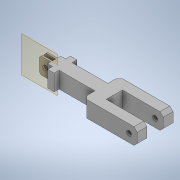
# Autodesk Inventor part: finger
Saved by Autodesk Inventor 2021 (Build 250183000, 183)
## iProperties
Created: 2020-11-29
Part Number: finger
Material: Generic
Document SubType Name: Modeling
Designer: awitc
Density: 1 g/cm^3
Appearance: Smooth - Medium Gray
Author: awitc
Autodesk Inventor part; units mm, degrees
ref_plane "YZ Plane" through (0, 0, 0) normal (1, 0, 0) x (0, 1, 0)
ref_plane "XZ Plane" through (0, 0, 0) normal (0, 1, 0) x (-1, 0, 0)
ref_plane "Work Plane1" through (0, 0, -10) normal (0, 0, 1) x (1, 0, 0)
sketch "Sketch12" plane through (0, 0, 0) normal (0, 1, 0) x (-1, 0, 0)
  line L0 (5, 4) -> (2, 4)
  line L1 (-2, 4) -> (-2, 7)
  line L2 (-2, 7) -> (2, 7)
  line L3 (2, 7) -> (2, 4)
  line L4 (6, 1) -> (12, 1)
  line L5 (12, -1) -> (6, -1)
  line L6 (12, -1) -> (6, -1)
  line L7 (6, -2) -> (12, -2)
  line L8 (5, -4) -> (5, 4)
  line L9 (12, -2) -> (12, -1)
  line L10 (12, 1) -> (12, 2)
  line L11 (12, 2) -> (6, 2)
  line L12 (6, -2) -> (5, -2)
  line L13 (6, -1) -> (5, -1)
  line L14 (6, 1) -> (5, 1)
  line L15 (6, 2) -> (5, 2)
  line L16 (-31, -11) -> (-57, -11)
  line L17 (-57, -11) -> (-57, -5)
  line L18 (-31, 11) -> (-57, 11)
  line L19 (-57, 11) -> (-57, 5)
  line L20 (-31, -11) -> (-24, -11)
  line L21 (-24, -11) -> (-24, -4)
  line L22 (-24, -4) -> (-24, 11)
  line L23 (-24, 11) -> (-31, 11)
  line L24 (-32, -4) -> (-32, 4)
  line L25 (-32, 4) -> (-32, 5)
  line L26 (-32, 5) -> (-57, 5)
  line L27 (-32, -4) -> (-32, -5)
  line L28 (-32, -5) -> (-57, -5)
  line L29 (5, -4) -> (2, -4)
  line L30 (2, -4) -> (2, -7)
  line L31 (2, -7) -> (-2, -7)
  line L32 (-2, -7) -> (-2, -4)
  line L33 (-2, -4) -> (-5, -4)
  line L34 (-5, -4) -> (-5, 4)
  line L35 (-5, 4) -> (-2, 4)
  line L36 (-5, 4) -> (-24, 4)
  line L37 (-5, -4) -> (-24, -4)
  point P0 (0, 0)
  point P1 (-31, 4)
  dimension "d118" = 4
  dimension "d156" = 7
  dimension "d170" = 3
  dimension "d171" = 3
  constraints: 76 end point, 14 perpendicular, 10 point on line, 4 horizontal, 4 vertical, 3 parallel, 1 collinear
  measures "d118" distance of L1.end L2.end
  measures "d156" distance of point (-31, 4) L18.start
  measures "d170" distance of L29.end L30.end
  measures "d171" distance of L32.end L33.end
ref_plane "Work Plane3" through (-12, 0, 2) normal (0, 0, 1) x (1, 0, 0)
extrude "Extrusion16" add sketch "Sketch12" along normal mid plane 10
extrude "Extrusion17" add sketch "Sketch12" along normal mid plane 8 contours L15 L11 L10 L4 L14 L8 | L13 L5 L9 L7 L12 L8
sketch "Sketch17" plane through (-12, 4, 2) normal (0, 0, 1) x (1, 0, 0)
  line L0 (7, -9) -> (7, 1) projected
  line L1 (7, -8) -> (3.5, -8)
  line L2 (0, -8) -> (7, -8) projected
  circle A0 centre (3.5, -4) radius 1.5
  point P0 (12, -4)
  point P1 (7, 0)
  dimension "d173" = 3
  constraints: 2 end point, 1 centre point, 1 midpoint
  measures "d173" diameter of A0
extrude "Extrusion18" cut sketch "Sketch17" against normal through all
extrude "Extrusion19" add sketch "Sketch12" along normal mid plane 6 contours L22 L21 L20 L16 L17 L28 L27 L24 L25 L26 L19 L18 L23
sketch "Sketch18" plane through (57, 3, -11) normal (0, 0, -1) x (-1, 0, 0)
  line L0 (0, -6) -> (0, 0) projected
  circle A0 centre (5, -3) radius 1.5
  point P0 (57, -3)
  dimension "d162" = 3
  constraints: 1 centre point
  measures "d162" diameter of A0
extrude "Extrusion20" cut sketch "Sketch18" against normal through all
chamfer "Chamfer12" distance 2 angle 45 6 edges at (57, 5, 8) (57, -5, 8) (57, 5, -8) (57, -5, -8) (24, 0, 11) (24, 0, -11)
chamfer "Chamfer13" distance 1 angle 45 4 edges at (-12, 5, 1.5) (-12, -5, 1.5) (-12, -5, -1.5) (-12, 5, -1.5)
body "Solid2"
